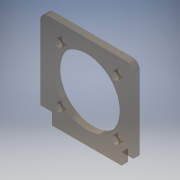
# Autodesk Inventor part: FanMount
Saved by Autodesk Inventor 2019 (Build 230136000, 136)
## iProperties
Created: 2019-01-17
Part Number: FanMount
Material: Polycarbonate, Smoke
Document SubType Name: Modeling
Designer: nxgam
Density: 1.2 g/cm^3
Appearance: Polycarbonate - Smoked
Author: nxgam
Autodesk Inventor part; units mm, degrees
ref_plane "YZ Plane" through (0, 0, 0) normal (1, 0, 0) x (0, 1, 0)
ref_plane "XZ Plane" through (0, 0, 0) normal (0, 1, 0) x (-1, 0, 0)
ref_plane "XY Plane" through (0, 0, 0) normal (0, 0, 1) x (1, 0, 0)
sketch "Sketch1" plane through (0, 0, 0) normal (0, 0, 1) x (1, 0, 0)
  line L0 (0, 0) -> (29.9974, 0)
  line L1 (29.9974, 0) -> (29.9974, 35.0774)
  line L2 (29.9974, 35.0774) -> (0, 35.0774)
  line L3 (0, 35.0774) -> (0, 0)
  line L4 (9.9187, 0) -> (20.0787, 0)
  dimension "d0" = 29.9974
  dimension "d1" = 35.0774
  dimension "d4" = 29.9974
  constraints: 10 end point, 2 horizontal, 2 parallel, 1 perpendicular, 1 point on line
  measures "d0" distance of L2.end L1.end
  measures "d1" distance of L1.end L0.end
  measures "d4" distance of L0.start L0.end
extrude "Extrusion1" add sketch "Sketch1" along normal blind 2.794
sketch "Sketch3" plane through (0, 0, 0) normal (0, 0, -1) x (-1, 0, 0)
  circle A0 centre (-27.16, 8.0774) radius 1.5875
  circle A1 centre (-2.84, 32.0774) radius 1.5875
  circle A2 centre (-27.16, 32.0774) radius 1.5875
  circle A3 centre (-2.84, 8.0774) radius 1.5875
  circle A4 centre (-15, 20.0774) radius 14.225
  line L0 (-30, 5.0774) -> (-30, 35.0774)
  line L1 (-30, 35.0774) -> (0, 35.0774)
  line L2 (0, 35.0774) -> (0, 5.0774)
  line L3 (0, 5.0774) -> (-30, 5.0774)
  point P0 (0, 0)
  constraints: 8 end point, 5 centre point, 2 horizontal, 2 vertical, 14 other
extrude "Extrusion2" cut sketch "Sketch3" against normal blind 2.794 contours A0 | A1 | A2 | A3 | A4
thicken "Thicken1" operation add thickness 5.08 both sides no extend neighbours yes toward (-1, 0, 0) faces at (0, 23.3849, 0.9313) (19.9983, 35.0774, 0.9313) (29.9974, 11.6925, 0.9313)
sketch "Sketch4" plane through (0, 0, 2.794) normal (0, 0, 1) x (1, 0, 0)
  circle A0 centre (2.84, 8.0774) radius 1.5875 projected
  circle A1 centre (2.84, 32.0774) radius 1.5875 projected
  circle A2 centre (27.16, 8.0774) radius 1.5875 projected
  circle A3 centre (27.16, 32.0774) radius 1.5875 projected
  circle A4 centre (15, 20.0774) radius 14.225 projected
  line L0 (-5.08, 0) -> (35.0774, 0) projected
  line L1 (35.0774, 0) -> (35.0774, 40.1574) projected
  line L2 (35.0774, 40.1574) -> (-5.08, 40.1574) projected
  line L3 (-5.08, 40.1574) -> (-5.08, 0) projected
  line L4 (-5.08, 0) -> (35.0774, 0) projected
  line L5 (-5.08, 0) -> (0, 0)
  line L6 (0, 0) -> (0, 5.08)
  line L7 (0, 5.08) -> (-5.08, 5.08)
  line L8 (-5.08, 5.08) -> (-5.08, 0)
  line L9 (35.0774, 0) -> (29.9974, 0)
  line L10 (29.9974, 0) -> (29.9974, 5.08)
  line L11 (29.9974, 5.08) -> (35.0774, 5.08)
  line L12 (35.0774, 5.08) -> (35.0774, 0)
  dimension "d12" = 5.08
  dimension "d13" = 5.08
  dimension "d14" = 5.08
  constraints: 16 end point, 4 parallel, 2 horizontal, 2 perpendicular, 1 point on line
  measures "d12" distance of L9.end L10.end
  measures "d13" distance of L10.end L11.end
  measures "d14" distance of L6.end L7.end
extrude "Extrusion3" cut sketch "Sketch4" against normal blind 25.4 contours L3 L7 L6 L0 | L10 L11 L1 L0
fillet "Fillet1" radius 3.175 2 edges at (35.0774, 40.1574, 1.397) (-5.08, 40.1574, 1.397)
equation "\"d13\" = d12"
equation "\"d14\" = d12"
body "Solid1"
